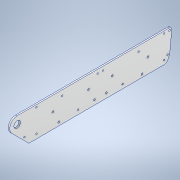
# Autodesk Inventor part: plyta_glowna
Saved by Autodesk Inventor 2020.3 (Build 243373000, 373)
## iProperties
Created: 2021-04-10
Part Number: plyta_glowna
Material: Aluminium 6061
Document SubType Name: Modeling
Designer: patryk.szydlik
Density: 2.7 g/cm^3
Appearance: Aluminium — płaski
Mass: 531.743 g
Surface Area: 1004.37 cm^2
Volume: 196.942 cm^3
Author: patryk.szydlik
Autodesk Inventor part; units mm, degrees
ref_plane "YZ Plane" through (0, 0, 0) normal (1, 0, 0) x (0, 1, 0)
ref_plane "XZ Plane" through (0, 0, 0) normal (0, 1, 0) x (-1, 0, 0)
ref_plane "XY Plane" through (0, 0, 0) normal (0, 0, 1) x (1, 0, 0)
sketch "Sketch2" plane through (0, 0, 0) normal (1, 0, 0) x (0, 1, 0)
  line L0 (127.2876, 96.9132) -> (-12.7124, 96.9132) construction
  line L1 (-12.7124, 96.9132) -> (-12.7124, -363.0868) construction
  line L2 (-12.7124, -363.0868) -> (127.2876, -363.0868) construction
  line L3 (127.2876, -363.0868) -> (127.2876, 96.9132) construction
  line L4 (97.2876, 66.9132) -> (17.2876, 66.9132) construction
  line L5 (17.2876, 66.9132) -> (17.2876, -333.0868) construction
  line L6 (17.2876, -333.0868) -> (97.2876, -333.0868) construction
  line L7 (97.2876, -333.0868) -> (97.2876, 66.9132) construction
  point P0 (0, 0)
  dimension "d2" = 140
  dimension "d3" = 460
  dimension "d4" = 80
  dimension "d5" = 400
  dimension "d6" = 30
  dimension "d7" = 30
  constraints: 16 end point, 4 parallel, 2 horizontal, 2 perpendicular
  measures "d2" distance of L2.end L1.end
  measures "d3" distance of L1.end L0.end
  measures "d4" distance of L6.end L5.end
  measures "d5" distance of L5.end L4.end
  measures "d6" distance between parallel lines of L3 L7
  measures "d7" distance between parallel lines of L0 L4
sketch "Sketch3" plane through (0, 0, 0) normal (1, 0, 0) x (0, 1, 0)
  circle A0 centre (-62.7124, 66.9132) radius 20
  line L0 (-12.7124, 96.9132) -> (-12.7124, -363.0868) construction
  circle A1 centre (-62.7124, -13.0868) radius 20
  circle A2 centre (-62.7124, -93.0868) radius 20
  circle A3 centre (-62.7124, -173.0868) radius 20
  circle A4 centre (-62.7124, -253.0868) radius 20
  circle A5 centre (-62.7124, -333.0868) radius 20
  line L1 (127.2876, 96.9132) -> (-12.7124, 96.9132) construction
  point P0 (0, 0)
  dimension "d8" = 40
  dimension "d9" = 50
  dimension "d12" = 80
  dimension "d17" = 30
  constraints: 6 centre point, 1 vertical, 10 other
  measures "d8" diameter of A0
  measures "d9" distance from line of L0 A0.centre
  measures "d12" distance of A0.centre A1.centre
  measures "d17" distance from line of A0.centre L1
sketch "Sketch1" plane through (0, 0, 0) normal (1, 0, 0) x (0, 1, 0)
  circle A0 centre (45.5719, 146.9132) radius 40
  circle A1 centre (85.5719, -453.0868) radius 40
  line L0 (127.2876, 96.9132) -> (-12.7124, 96.9132) construction
  line L1 (-12.7124, -363.0868) -> (127.2876, -363.0868) construction
  line L2 (-62.7124, 66.9132) -> (-62.7124, -13.0868) construction
  line L3 (-62.7124, -253.0868) -> (-62.7124, -333.0868) construction
  line L4 (85.2399, 141.7706) -> (125.4799, -450.3748) construction
  circle A2 centre (-62.7124, 66.9132) radius 20 projected
  line L5 (17.2876, 175.1975) -> (-76.8545, 81.0553)
  circle A3 centre (-62.7124, -333.0868) radius 20 projected
  line L6 (-76.8545, -347.2289) -> (57.2876, -481.3711) construction
  point P0 (0, 0)
  dimension "d0" = 80
  dimension "d1" = 80
  dimension "d18" = 50
  dimension "d19" = 90
  dimension "d45" = 135
  dimension "d46" = 135
  constraints: 10 end point, 4 point on circle, 3 tangent, 2 centre point, 2 coincident, 2 vertical, 6 other
  measures "d0" diameter of A0
  measures "d1" diameter of A1
  measures "d18" distance from line of A0.centre L0
  measures "d19" distance from line of A1.centre L1
  measures "d45" angle of L2 L5
  measures "d46" angle of L3 L6
sketch "Sketch4" plane through (0, 0, 0) normal (1, 0, 0) x (0, 1, 0)
  line L0 (37.6815, -3.0868) -> (-57.7124, 26.9132) construction
  circle A0 centre (-62.7124, 66.9132) radius 20 projected
  circle A1 centre (-62.7124, -13.0868) radius 20 projected
  line L1 (-62.7124, 66.9132) -> (-62.7124, -13.0868) construction
  circle A2 centre (-27.7124, 112.5679) radius 20 construction
  circle A3 centre (-27.7124, 32.5679) radius 20 construction
  line L2 (-27.7124, 72.5679) -> (37.6815, -3.0868) construction
  line L3 (-27.7124, 72.5679) -> (-57.7124, 26.9132) construction
  line L4 (37.6815, -3.0868) -> (-42.7124, 49.7406) construction
  line L5 (-12.7124, 96.9132) -> (-12.7124, -363.0868) construction
  point P0 (0, 0)
  point P1 (-61.7124, 47.9132)
  point P2 (83.0715, 79.9132)
  point P3 (83.0715, -80.0868)
  point P4 (37.6815, -163.0868)
  point P5 (83.0715, -240.0868)
  point P6 (37.6815, -323.0868)
  dimension "d22" = 40
  dimension "d23" = 5
  dimension "d24" = 30
  dimension "d25" = 40
  dimension "d26" = 40
  dimension "d27" = 80
  dimension "d28" = 40
  dimension "d29" = 100
  dimension "d30" = 100
  dimension "d31" = 35
  dimension "d32" = 54.6292
  dimension "d33" = 27.3146
  dimension "d34" = 56.691
  dimension "d35" = 95.3939
  dimension "d36" = 45.39
  dimension "d37" = 83
  dimension "d40" = 160
  constraints: 8 end point, 2 centre point, 2 vertical alignment, 1 coincident, 1 midpoint, 1 vertical, 4 other
  measures "d22" vertical distance of point (-62.712, 66.913) L0.end
  measures "d23" horizontal distance of point (-62.712, 66.913) L0.end
  measures "d24" vertical distance of L0.end L0.start
  measures "d25" diameter of A3
  measures "d26" diameter of A2
  measures "d27" distance of A3.centre A2.centre
  measures "d28" distance of A3.centre L2.start
  measures "d29" distance of L0.start L0.end
  measures "d30" distance of L2.start L0.start
  measures "d31" horizontal distance of point (-62.712, 66.913) A2.centre
  measures "d32" distance of L0.end L2.start
  measures "d33" distance of L0.end L4.end
  measures "d34" angle of L5 L4
  measures "d35" horizontal distance of L0.end L0.start
  measures "d36" horizontal distance of L0.start point (83.072, 79.913)
  measures "d37" vertical distance of L0.start point (83.072, 79.913)
  measures "d40" distance of point (83.072, 79.913) point (83.072, -80.087)
sketch "Sketch6" plane through (0, 0, 0) normal (1, 0, 0) x (0, 1, 0)
  line L0 (234.6261, -208.0868) -> (-157.479, -208.0868) construction
  line L1 (237.7494, -58.0868) -> (-154.3557, -58.0868) construction
  line L2 (17.2876, -333.0868) -> (97.2876, -333.0868) construction
  line L3 (97.2876, 66.9132) -> (17.2876, 66.9132) construction
  point P0 (0, 0)
  dimension "d61" = 125
  dimension "d62" = 125
  constraints: 4 end point, 2 horizontal
  measures "d61" distance between parallel lines of L1 L3
  measures "d62" distance between parallel lines of L2 L0
sketch "Sketch5" plane through (0, 0, 0) normal (1, 0, 0) x (0, 1, 0)
  arc A0 (90.5716, 146.9132) -> (47.894, 164.5909) centre (65.5716, 146.9132) ccw
  arc A1 (47.894, 164.5909) -> (90.5716, 146.9132) centre (65.5716, 146.9132) ccw construction
  line L0 (114.7874, 96.9132) -> (-25.2126, 96.9132) construction
  line L1 (-32.7126, -363.0868) -> (107.2874, -363.0868) construction
  line L2 (217.7491, -58.0868) -> (-174.356, -58.0868) construction
  line L3 (214.6258, -208.0868) -> (-177.4793, -208.0868) construction
  circle A2 centre (65.5716, 146.9132) radius 11
  circle A3 centre (65.5716, 146.9132) radius 55 construction
  line L4 (-9.4284, 107.2685) -> (47.894, 164.5909)
  line L5 (-2.7126, 66.9132) -> (-2.7126, -333.0868) construction
  line L6 (-62.7124, -13.0868) -> (-62.7124, -93.0868) construction
  line L7 (-62.7124, -173.0868) -> (-62.7124, -253.0868) construction
  line L8 (90.5716, -363.0868) -> (90.5716, 146.9132)
  line L9 (90.5716, -363.0868) -> (90.5716, -366.2493)
  arc A4 (82.3188, -373.7114) -> (90.5716, -366.2493) centre (83.0716, -366.2493) ccw
  arc A5 (12.4757, -366.2343) -> (14.9188, -366.9114) centre (15.6716, -359.4493) ccw
  line L10 (82.3188, -373.7114) -> (14.9188, -366.9114)
  arc A6 (-7.9036, -348.1319) -> (-0.1706, -360.2774) centre (5.5716, -348.0868) ccw
  line L11 (12.4757, -366.2343) -> (-0.1706, -360.2774)
  line L12 (-7.9036, -348.1319) -> (-9.4284, 107.2685)
  point P0 (0, 0)
  point P1 (83.0716, 81.9132)
  point P2 (83.0716, -348.0868)
  point P3 (16.3276, 122.4179)
  point P4 (8.0719, -82.4742)
  point P5 (8.0719, -243.0868)
  point P6 (-17.7126, -58.0868)
  point P7 (-17.7126, -208.0868)
  point P8 (5.5716, 81.9132)
  point P9 (-62.7124, 66.9132)
  point P10 (-62.7124, -333.0868)
  point P11 (-62.7124, -53.0868)
  point P12 (-62.7124, -213.0868)
  point P13 (2.2876, 6.9132)
  point P14 (42.2876, 26.9132)
  point P15 (47.2876, -93.0868)
  point P16 (7.2876, -113.0868)
  point P17 (7.2876, -153.0868)
  point P18 (47.2876, -173.0868)
  point P19 (42.2876, -293.0868)
  point P20 (2.2876, -273.0868)
  point P21 (2.2876, 6.9132)
  point P22 (-62.7124, 66.9132)
  point P23 (5.5716, -208.0868)
  point P24 (5.5716, -58.0868)
  point P25 (73.0216, -4.2568)
  point P26 (78.0216, -124.2568)
  point P27 (78.0216, -141.9168)
  point P28 (73.0216, -261.9168)
  dimension "d84" = 110
  dimension "d47" = 50
  dimension "d63" = 15
  dimension "d65" = 15
  dimension "d81" = 22
  dimension "d101" = 7.5
  dimension "d151" = 15
  dimension "d155" = 15
  dimension "d159" = 15
  dimension "d163" = 60
  dimension "d164" = 65
  dimension "d165" = 20
  dimension "d166" = 40
  dimension "d174" = 60
  dimension "d175" = 70
  dimension "d176" = 40
  dimension "d177" = 20
  dimension "d196" = 128.284
  dimension "d198" = 11.17
  dimension "d199" = 70.734
  dimension "d200" = 11.17
  dimension "d201" = 70.734
  dimension "d204" = 11.17
  dimension "d213" = 65
  dimension "d214" = 40
  dimension "d215" = 20
  dimension "d216" = 20
  dimension "d217" = 40
  dimension "d218" = 70.734
  dimension "d219" = 70.734
  dimension "d220" = 11.17
  dimension "d221" = 67.4
  dimension "d222" = 6.8
  dimension "d223" = 7.5
  dimension "d224" = 15
  dimension "d225" = 15
  constraints: 26 end point, 10 point on circle, 7 coincident, 6 centre point, 5 point on line, 5 tangent, 2 midpoint, 1 horizontal alignment, 1 vertical, 1 vertical alignment, 3 other
  measures "d47" diameter of A0
  measures "d63" distance from line of L0 point (83.072, 81.913)
  measures "d65" distance from line of L1 point (83.072, -348.087)
  measures "d81" diameter of A2
  measures "d101" distance from line of point (16.328, 122.418) L4
  measures "d151" distance from line of L5 point (-17.713, -58.087)
  measures "d155" distance from line of L5 point (-17.713, -208.087)
  measures "d159" distance from line of L0 point (5.572, 81.913)
  measures "d163" vertical distance of point (-62.712, 66.913) point (2.288, 6.913)
  measures "d164" horizontal distance of point (-62.712, 66.913) point (2.288, 6.913)
  measures "d165" vertical distance of point (2.288, 6.913) point (42.288, 26.913)
  measures "d166" horizontal distance of point (2.288, 6.913) point (42.288, 26.913)
  measures "d174" vertical distance of point (-62.712, -213.087) point (7.288, -153.087)
  measures "d175" horizontal distance of point (-62.712, -213.087) point (7.288, -153.087)
  measures "d176" horizontal distance of point (47.288, -173.087) point (7.288, -153.087)
  measures "d177" vertical distance of point (47.288, -173.087) point (7.288, -153.087)
  measures "d196" horizontal distance of point (65.572, 146.913) point (-62.712, 66.913)
  measures "d198" vertical distance of point (73.022, -4.257) point (2.288, 6.913)
  measures "d199" horizontal distance of point (2.288, 6.913) point (73.022, -4.257)
  measures "d200" vertical distance of point (7.288, -113.087) point (78.022, -124.257)
  measures "d201" horizontal distance of point (7.288, -113.087) point (78.022, -124.257)
  measures "d204" vertical distance of point (2.288, -273.087) point (73.022, -261.917)
  measures "d213" horizontal distance of point (2.288, -273.087) L7.end
  measures "d214" horizontal distance of point (2.288, -273.087) point (42.288, -293.087)
  measures "d215" vertical distance of point (2.288, -273.087) point (42.288, -293.087)
  measures "d216" vertical distance of point (7.288, -113.087) point (47.288, -93.087)
  measures "d217" horizontal distance of point (47.288, -93.087) point (7.288, -113.087)
  measures "d218" horizontal distance of point (7.288, -153.087) point (78.022, -141.917)
  measures "d219" horizontal distance of point (2.288, -273.087) point (73.022, -261.917)
  measures "d220" vertical distance of point (7.288, -153.087) point (78.022, -141.917)
  measures "d221" horizontal distance of point (15.672, -359.449) point (83.072, -366.249)
  measures "d222" vertical distance of point (15.672, -359.449) point (83.072, -366.249)
  measures "d223" distance from line of L8 point (83.072, -366.249)
  measures "d224" diameter of A4
  measures "d225" diameter of A5
extrude "Extrusion1" add sketch "Sketch5" against normal blind 5
hole "Hole1" at (0, 83.0716, 81.9132) at (0, 16.3276, 122.4179) at (0, 5.5716, -348.0868) at (0, 83.0716, -348.0868) at (0, -17.7126, -58.0868) at (0, -17.7126, -208.0868) at (0, 5.5716, 81.9132) at (0, 5.5716, -58.0868) at (0, 5.5716, -208.0868) direction (-1, 0, 0) diameter 5 end through all clearance for "Flat Head Machine Screw" size "M5" standard "Ansi Metric M Profile"
hole "Otwór2" at (0, 2.2876, 6.9132) at (0, 42.2876, 26.9132) at (0, 7.2876, -113.0868) at (0, 47.2876, -93.0868) at (0, 7.2876, -153.0868) at (0, 47.2876, -173.0868) at (0, 2.2876, -273.0868) at (0, 42.2876, -293.0868) at (0, 83.0716, -366.2493) direction (-1, 0, 0) diameter 6 end through all
hole "Otwór3" at (0, 73.0216, -4.2568) at (0, 78.0216, -141.9168) at (0, 78.0216, -124.2568) at (0, 73.0216, -261.9168) at (0, 15.6716, -359.4493) direction (-1, 0, 0) diameter 5 end through all
equation "\"d28\" = 0.5 * d27"
equation "\"d30\" = d29"
equation "\"d33\" = 0.5 * d32"
equation "\"d62\" = d61"
body "Solid1"
